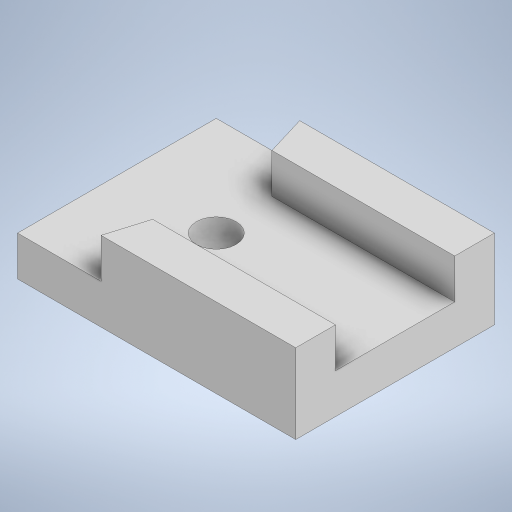
# Autodesk Inventor part: Стенка
Saved by Autodesk Inventor 2023 (Build 270158000, 158)
## iProperties
Created: 2022-04-28
Part Number: Стенка
Material: Типовые
Document SubType Name: Modeling
Designer: User
Density: 1 g/cm^3
Appearance: По умолчанию
Author: User
Autodesk Inventor part; units mm, degrees
ref_plane "YZ Plane" through (0, 0, 0) normal (1, 0, 0) x (0, 1, 0)
ref_plane "XZ Plane" through (0, 0, 0) normal (0, 1, 0) x (-1, 0, 0)
ref_plane "XY Plane" through (0, 0, 0) normal (0, 0, 1) x (1, 0, 0)
sketch "Эскиз1" plane through (0, 0, 0) normal (0, 1, 0) x (-1, 0, 0)
  line L0 (0, 0) -> (70, 0)
  line L1 (70, 0) -> (70, -50)
  line L2 (70, -50) -> (0, -50)
  line L3 (0, -50) -> (0, 0)
  dimension "d0" = 70
  dimension "d1" = 50
  constraints: 8 end point, 2 parallel, 1 horizontal, 1 perpendicular
  measures "d0" distance of L1.end L2.end
  measures "d1" distance of L0.end L1.end
extrude "Выдавливание1" add sketch "Эскиз1" along normal blind 10
sketch "Эскиз2" plane through (0, 10, 0) normal (0, 1, 0) x (1, 0, 0)
  line L0 (0, 0) -> (0, 50) projected
  line L1 (0, 25) -> (-45, 25)
  circle A0 centre (-45, 25) radius 5
  line L2 (0, 25) -> (0, 40)
  line L3 (0, 40) -> (-46, 40)
  line L4 (0, 25) -> (0, 10)
  line L5 (0, 10) -> (-46, 10)
  line L6 (-45, 25) -> (-70, 25)
  line L7 (-70, 50) -> (-70, 0) projected
  line L8 (-45, 25) -> (5, 25) construction
  line L9 (-45, 25) -> (-52.4371, 0.2096)
  line L10 (-45, 25) -> (15, 25) construction
  line L11 (-52.4371, 0.2096) -> (-52.4371, 49.7904)
  line L12 (-45, 25) -> (-52.4371, 49.7904)
  circle A1 centre (-45, 25) radius 9
  line L13 (-46, 40) -> (-49, 50)
  line L14 (-46, 10) -> (-49, 0)
  line L15 (-49, 0) -> (0, 0)
  line L16 (0, 0) -> (0, 50)
  line L17 (0, 50) -> (-49, 50)
  dimension "d4" = 45
  dimension "d5" = 10
  dimension "d6" = 15
  dimension "d7" = 15
  dimension "d12" = 146.602
  dimension "d13" = 18
  dimension "d18" = 49
  dimension "d19" = 46
  constraints: 32 end point, 4 perpendicular, 3 horizontal, 2 centre point, 2 coincident, 2 equal length, 2 midpoint, 2 parallel, 2 point on line, 1 vertical
  measures "d4" distance of L1.start L1.end
  measures "d5" diameter of A0
  measures "d6" distance of L1.start L2.end
  measures "d7" distance of L1.start L4.end
  measures "d12" angle of L9 L12
  measures "d13" diameter of A1
  measures "d18" distance of L0.end L13.end
  measures "d19" distance of L2.end L3.end
extrude "Выдавливание2" add sketch "Эскиз2" along normal blind 10 contours L15 L14 L5 L0 | L3 L13 L17 L0
extrude "Выдавливание3" cut sketch "Эскиз2" against normal blind 42.5 contours A0 L9 L1 | L1 L12 A0 | L9 A0 L6 | L6 A0 L12
